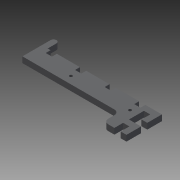
# Autodesk Inventor part: spoolHolder_a
Saved by Autodesk Inventor 2013 (Build 170138000, 138)
## iProperties
Created: 2015-01-14
Part Number: spoolHolder_a
Material: Generic
Document SubType Name: Modeling
Designer: dzban
Density: 1 g/cm^3
Author: dzban
Autodesk Inventor part; units mm, degrees
ref_plane "YZ Plane" through (0, 0, 0) normal (1, 0, 0) x (0, 1, 0)
ref_plane "XZ Plane" through (0, 0, 0) normal (0, 1, 0) x (-1, 0, 0)
ref_plane "XY Plane" through (0, 0, 0) normal (0, 0, 1) x (1, 0, 0)
sketch "Sketch1" plane through (0, 0, 0) normal (0, 0, 1) x (1, 0, 0)
  arc A0 (11.7049, -23.2932) -> (16.7049, -28.2932) centre (16.7049, -23.2932) ccw
  line L0 (16.7049, -28.2932) -> (23.1049, -28.2932)
  line L1 (23.1049, -28.2932) -> (23.1049, -19.2932)
  line L2 (23.1049, -19.2932) -> (29.5049, -19.2932)
  line L3 (29.5049, -19.2932) -> (29.5049, -28.2932)
  line L4 (29.5049, -28.2932) -> (35.5049, -28.2932)
  line L5 (35.5049, -28.2932) -> (35.5049, -13.2932)
  line L6 (35.5049, -13.2932) -> (23.1049, -13.2932)
  line L7 (23.1049, -13.2932) -> (23.1049, 2.1068)
  line L8 (23.1049, 2.1068) -> (29.5049, 2.1068)
  line L9 (29.5049, 2.1068) -> (29.5049, -6.8932)
  line L10 (29.5049, -6.8932) -> (35.5049, -6.8932)
  line L11 (35.5049, -6.8932) -> (35.5049, 8.1068)
  line L12 (35.5049, 8.1068) -> (18.5049, 8.1068)
  line L13 (18.5049, 8.1068) -> (18.5049, 3.1068)
  line L14 (18.5049, 3.1068) -> (12.1049, 3.1068)
  line L15 (12.1049, 3.1068) -> (12.1049, 8.1068)
  line L16 (12.1049, 8.1068) -> (-11.8951, 8.1068)
  line L17 (-11.8951, 8.1068) -> (-11.8951, 3.1068)
  line L18 (-11.8951, 3.1068) -> (-18.2951, 3.1068)
  line L19 (-18.2951, 3.1068) -> (-18.2951, 8.1068)
  line L20 (-18.2951, 8.1068) -> (-42.2951, 8.1068)
  line L21 (-42.2951, 8.1068) -> (-42.2951, 3.1068)
  line L22 (-42.2951, 3.1068) -> (-48.6951, 3.1068)
  line L23 (-48.6951, 3.1068) -> (-48.6951, 8.1068)
  line L24 (-48.6951, 8.1068) -> (-72.4951, 8.1068)
  line L25 (-72.4951, 8.1068) -> (-72.4951, 3.1068)
  line L26 (-72.4951, 3.1068) -> (-78.8951, 3.1068)
  line L27 (-78.8951, 3.1068) -> (-78.8951, 8.1068)
  line L28 (-78.8951, 8.1068) -> (-81.8951, 8.1068)
  line L29 (-81.8951, 8.1068) -> (-81.8951, 17.1068)
  arc A1 (-81.8951, 17.1068) -> (-87.8951, 17.1068) centre (-84.8951, 17.1068) ccw
  line L30 (-87.8951, 17.1068) -> (-87.8951, -11.8932)
  line L31 (-87.8951, -11.8932) -> (6.7049, -11.8932)
  arc A2 (11.7049, -16.8932) -> (6.7049, -11.8932) centre (6.7049, -16.8932) ccw
  line L32 (11.7049, -16.8932) -> (11.7049, -23.2932)
  circle A3 centre (-45.4951, -4.3932) radius 1.5
  circle A4 centre (15.3049, -4.3932) radius 1.5
  point P0 (0, 0)
  constraints: 66 end point, 6 point on circle, 5 centre point
extrude "Extrusion1" add sketch "Sketch1" along normal blind 6
body "Solid1"
